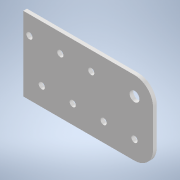
# Autodesk Inventor part: fixation_plate2
Saved by Autodesk Inventor 2022 (Build 260153000, 153)
## iProperties
Created: 2022-01-31
Part Number: fixation_plate2
Material: Generic
Document SubType Name: Modeling
Designer: Martijn
Density: 1 g/cm^3
Appearance: Default
Author: Martijn
Autodesk Inventor part; units mm, degrees
ref_plane "YZ Plane" through (0, 0, 0) normal (1, 0, 0) x (0, 1, 0)
ref_plane "XZ Plane" through (0, 0, 0) normal (0, 1, 0) x (-1, 0, 0)
ref_plane "XY Plane" through (0, 0, 0) normal (0, 0, 1) x (1, 0, 0)
sketch "Sketch1" plane through (0, 0, 0) normal (0, 0, 1) x (1, 0, 0)
  line L0 (0, 30) -> (85, 30)
  circle A0 centre (5, 15) radius 2.5
  circle A1 centre (30, 15) radius 2.5
  circle A2 centre (85, 15) radius 4
  circle A3 centre (55, 15) radius 2.5
  line L1 (0, 30) -> (0, -30)
  line L2 (0, -30) -> (85, -30)
  arc A4 (85, -30) -> (100, -15) centre (85, -15) ccw
  arc A5 (100, 15) -> (85, 30) centre (85, 15) ccw
  line L3 (100, 15) -> (100, -15)
  line L4 (0, -46.3492) -> (0, 46.3492) projected
  circle A6 centre (60, -15) radius 2.5
  circle A7 centre (35, -15) radius 2.5
  circle A8 centre (10, -15) radius 2.5
  circle A9 centre (85, -15) radius 2.5
  point P0 (0, 0)
  dimension "d2" = 5
  dimension "d6" = 8
  dimension "d12" = 25
  dimension "d13" = 25
  dimension "d14" = 60
  dimension "d15" = 30
  dimension "d16" = 15
  dimension "d17" = 15
  dimension "d18" = 5
  dimension "d20" = 15
  dimension "d21" = 85
  dimension "d22" = 15
  dimension "d23" = 15
  dimension "d24" = 25
  dimension "d25" = 25
  dimension "d26" = 25
  dimension "d27" = 15
  dimension "d28" = 15
  dimension "d29" = 15
  constraints: 10 centre point, 8 end point, 6 equal radius, 4 point on circle, 4 tangent, 3 perpendicular, 2 coincident, 1 collinear, 1 vertical
  measures "d2" diameter of A0
  measures "d6" diameter of A2
  measures "d12" distance of A1.centre A3.centre
  measures "d13" distance of A1.centre A0.centre
  measures "d14" distance of L0.start L1.end
  measures "d15" distance from line of L0 point (0, 0)
  measures "d16" distance from line of L0 A1.centre
  measures "d17" distance from line of L0 A0.centre
  measures "d18" distance from line of L1 A0.centre
  measures "d20" radius of A4
  measures "d21" distance from line of L1 A2.centre
  measures "d22" distance from line of L0 A2.centre
  measures "d23" distance from line of L0 A3.centre
  measures "d24" distance of A4.centre A6.centre
  measures "d25" distance of A6.centre A7.centre
  measures "d26" distance of A7.centre A8.centre
  measures "d27" distance from line of L2 A6.centre
  measures "d28" distance from line of L2 A7.centre
  measures "d29" distance from line of L2 A8.centre
extrude "Extrusion1" add sketch "Sketch1" along normal blind 3
body "Solid1"
